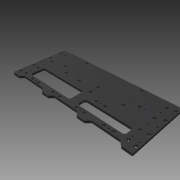
# Autodesk Inventor part: front
Saved by Autodesk Inventor 2014 (Build 180170000, 170)
## iProperties
Created: 2013-12-05
Part Number: front
Material: Plywood, Finish
Document SubType Name: Modeling
Designer: buben
Density: 0.552 g/cm^3
Appearance: Plywood - New
Author: buben
Subject: Laser Cutted
Autodesk Inventor part; units mm, degrees
ref_plane "YZ Plane" through (0, 0, 0) normal (1, 0, 0) x (0, 1, 0)
ref_plane "XZ Plane" through (0, 0, 0) normal (0, 1, 0) x (-1, 0, 0)
ref_plane "XY Plane" through (0, 0, 0) normal (0, 0, 1) x (1, 0, 0)
sketch "Sketch1" plane through (0, 0, 0) normal (0, 0, 1) x (1, 0, 0)
  line L0 (0, 0) -> (355, 0)
  line L1 (355, 0) -> (355, 150)
  line L2 (355, 150) -> (0, 150)
  line L3 (0, 150) -> (0, 0)
  dimension "d0" = 150
  dimension "d1" = 355
  constraints: 8 end point, 2 parallel, 1 horizontal, 1 perpendicular
  measures "d0" distance of L2.end L0.start
  measures "d1" distance of L0.start L0.end
extrude "Extrusion1" add sketch "Sketch1" along normal blind 6.5
sketch "Sketch3" plane through (0, 0, 6.5) normal (0, 0, 1) x (1, 0, 0)
  line L0 (0, 0) -> (355, 0) projected
  line L1 (355, 150) -> (0, 150) projected
  line L2 (0, 150) -> (0, 0) projected
  circle A0 centre (64.5, 96) radius 4
  circle A1 centre (290.5, 96) radius 4
  line L3 (64.5, 96) -> (290.5, 96) construction
  point P0 (177.5, 96)
  point P1 (177.5, 150)
  dimension "d9" = 8
  dimension "d10" = 96
  dimension "d11" = 226
  constraints: 2 centre point, 2 end point, 2 midpoint, 1 equal radius, 1 horizontal alignment, 1 perpendicular, 1 vertical alignment
  measures "d9" diameter of A0
  measures "d10" distance from line of L0 L3.start
  measures "d11" distance of L3.start L3.end
extrude "Extrusion3" cut sketch "Sketch3" against normal through all
sketch "Sketch4" plane through (0, 0, 6.5) normal (0, 0, 1) x (1, 0, 0)
  line L0 (0, 0) -> (355, 0) projected
  line L1 (355, 150) -> (0, 150) projected
  line L2 (0, 150) -> (0, 0) projected
  circle A0 centre (6.25, 18.5) radius 2.25
  circle A1 centre (6.25, 70.5) radius 2.25
  circle A2 centre (6.25, 122.5) radius 2.25
  line L3 (177.5, 150) -> (177.5, 0) construction
  line L4 (3, 138) -> (9.5, 138)
  line L5 (9.5, 138) -> (9.5, 130)
  line L6 (9.5, 130) -> (3, 130)
  line L7 (3, 130) -> (3, 138)
  line L8 (3, 100.5) -> (9.5, 100.5)
  line L9 (9.5, 100.5) -> (9.5, 92.5)
  line L10 (9.5, 92.5) -> (3, 92.5)
  line L11 (3, 92.5) -> (3, 100.5)
  line L12 (3, 48.5) -> (9.5, 48.5)
  line L13 (9.5, 48.5) -> (9.5, 40.5)
  line L14 (9.5, 40.5) -> (3, 40.5)
  line L15 (3, 40.5) -> (3, 48.5)
  line L16 (3, 11) -> (9.5, 11)
  line L17 (9.5, 11) -> (9.5, 3)
  line L18 (9.5, 3) -> (3, 3)
  line L19 (3, 3) -> (3, 11)
  line L20 (6.25, 18.5) -> (6.25, 70.5) construction
  line L21 (6.25, 70.5) -> (6.25, 122.5) construction
  circle A3 centre (348.75, 18.5) radius 2.25
  circle A4 centre (348.75, 70.5) radius 2.25
  circle A5 centre (348.75, 122.5) radius 2.25
  line L22 (352, 138) -> (345.5, 138)
  line L23 (345.5, 138) -> (345.5, 130)
  line L24 (345.5, 130) -> (352, 130)
  line L25 (352, 130) -> (352, 138)
  line L26 (352, 100.5) -> (345.5, 100.5)
  line L27 (345.5, 100.5) -> (345.5, 92.5)
  line L28 (345.5, 92.5) -> (352, 92.5)
  line L29 (352, 92.5) -> (352, 100.5)
  line L30 (352, 48.5) -> (345.5, 48.5)
  line L31 (345.5, 48.5) -> (345.5, 40.5)
  line L32 (345.5, 40.5) -> (352, 40.5)
  line L33 (352, 40.5) -> (352, 48.5)
  line L34 (352, 11) -> (345.5, 11)
  line L35 (345.5, 11) -> (345.5, 3)
  line L36 (345.5, 3) -> (352, 3)
  line L37 (352, 3) -> (352, 11)
  line L38 (348.75, 18.5) -> (348.75, 70.5) construction
  line L39 (348.75, 70.5) -> (348.75, 122.5) construction
  point P0 (6.25, 130)
  point P1 (3, 44.5)
  point P2 (6.25, 44.5)
  point P3 (3, 96.5)
  point P4 (6.25, 96.5)
  point P5 (348.75, 130)
  point P6 (352, 44.5)
  point P7 (348.75, 44.5)
  point P8 (352, 96.5)
  point P9 (348.75, 96.5)
  dimension "d14" = 18.5
  dimension "d15" = 52
  dimension "d16" = 52
  dimension "d17" = 4.5
  dimension "d18" = 6.5
  dimension "d19" = 8
  dimension "d20" = 8
  dimension "d21" = 8
  dimension "d22" = 8
  dimension "d28" = 3
  dimension "d90" = 7.5
  dimension "d91" = 7.5
  constraints: 74 end point, 24 symmetric about line, 9 parallel, 7 collinear, 7 midpoint, 6 centre point, 4 horizontal, 4 perpendicular, 3 vertical alignment, 2 equal radius, 2 horizontal alignment, 3 other
  measures "d14" distance from line of L0 L20.start
  measures "d15" distance of L20.start L20.end
  measures "d16" distance of L20.end L21.end
  measures "d17" diameter of A0
  measures "d18" distance of L4.start L4.end
  measures "d19" distance of L6.end L4.start
  measures "d20" distance of L10.end L8.start
  measures "d21" distance of L14.end L12.start
  measures "d22" distance of L18.end L16.start
  measures "d28" distance between parallel lines of L2 L7
  measures "d90" distance from line of L21.end L6
  measures "d91" distance from line of L20.start L16
extrude "Extrusion4" cut sketch "Sketch4" against normal through all
sketch "Sketch5" plane through (0, 0, 6.5) normal (0, 0, 1) x (1, 0, 0)
  line L0 (0, 0) -> (355, 0) projected
  line L1 (51, 9.5) -> (59, 9.5)
  line L2 (59, 9.5) -> (59, 3)
  line L3 (59, 3) -> (51, 3)
  line L4 (51, 3) -> (51, 9.5)
  line L5 (74, 9.5) -> (82, 9.5)
  line L6 (82, 9.5) -> (82, 3)
  line L7 (82, 3) -> (74, 3)
  line L8 (74, 3) -> (74, 9.5)
  line L9 (59, 9.5) -> (74, 3) construction
  line L10 (74, 9.5) -> (59, 3) construction
  circle A0 centre (66.5, 6.25) radius 2.25
  line L11 (125, 9.5) -> (133, 9.5)
  line L12 (133, 9.5) -> (133, 3)
  line L13 (133, 3) -> (125, 3)
  line L14 (125, 3) -> (125, 9.5)
  line L15 (148, 9.5) -> (156, 9.5)
  line L16 (156, 9.5) -> (156, 3)
  line L17 (156, 3) -> (148, 3)
  line L18 (148, 3) -> (148, 9.5)
  line L19 (133, 9.5) -> (148, 3) construction
  line L20 (148, 9.5) -> (133, 3) construction
  circle A1 centre (140.5, 6.25) radius 2.25
  line L21 (199, 9.5) -> (207, 9.5)
  line L22 (207, 9.5) -> (207, 3)
  line L23 (207, 3) -> (199, 3)
  line L24 (199, 3) -> (199, 9.5)
  line L25 (222, 9.5) -> (230, 9.5)
  line L26 (230, 9.5) -> (230, 3)
  line L27 (230, 3) -> (222, 3)
  line L28 (222, 3) -> (222, 9.5)
  line L29 (207, 9.5) -> (222, 3) construction
  line L30 (222, 9.5) -> (207, 3) construction
  circle A2 centre (214.5, 6.25) radius 2.25
  line L31 (273, 9.5) -> (281, 9.5)
  line L32 (281, 9.5) -> (281, 3)
  line L33 (281, 3) -> (273, 3)
  line L34 (273, 3) -> (273, 9.5)
  line L35 (296, 9.5) -> (304, 9.5)
  line L36 (304, 9.5) -> (304, 3)
  line L37 (304, 3) -> (296, 3)
  line L38 (296, 3) -> (296, 9.5)
  line L39 (281, 9.5) -> (296, 3) construction
  line L40 (296, 9.5) -> (281, 3) construction
  circle A3 centre (288.5, 6.25) radius 2.25
  line L41 (82, 6.25) -> (125, 6.25) construction
  line L42 (156, 6.25) -> (199, 6.25) construction
  line L43 (230, 6.25) -> (273, 6.25) construction
  line L44 (9.5, 11) -> (9.5, 3) projected
  line L45 (345.5, 3) -> (345.5, 11) projected
  point P0 (288.5, 6.25)
  dimension "d31" = 8
  dimension "d32" = 6.5
  dimension "d33" = 8
  dimension "d34" = 15
  dimension "d35" = 4.5
  dimension "d36" = 8
  dimension "d37" = 6.5
  dimension "d38" = 8
  dimension "d39" = 15
  dimension "d40" = 4.5
  dimension "d41" = 8
  dimension "d42" = 6.5
  dimension "d43" = 8
  dimension "d44" = 15
  dimension "d45" = 4.5
  dimension "d46" = 8
  dimension "d47" = 6.5
  dimension "d48" = 8
  dimension "d49" = 15
  dimension "d50" = 4.5
  dimension "d51" = 3
  dimension "d88" = 57
  dimension "d89" = 57
  constraints: 86 end point, 16 parallel, 11 midpoint, 10 collinear, 8 horizontal, 8 perpendicular, 4 centre point, 3 horizontal alignment
  measures "d31" distance of L1.start L1.end
  measures "d32" distance of L3.end L1.start
  measures "d33" distance of L5.start L5.end
  measures "d34" distance between parallel lines of L8 L2
  measures "d35" diameter of A0
  measures "d36" distance of L14.end L11.end
  measures "d37" distance of L14.start L14.end
  measures "d38" distance of L20.start L15.end
  measures "d39" distance between parallel lines of L18 L12
  measures "d40" diameter of A1
  measures "d41" distance of L24.end L21.end
  measures "d42" distance of L24.start L24.end
  measures "d43" distance of L30.start L25.end
  measures "d44" distance between parallel lines of L28 L22
  measures "d45" diameter of A2
  measures "d46" distance of L34.end L31.end
  measures "d47" distance of L34.start L34.end
  measures "d48" distance of L40.start L35.end
  measures "d49" distance between parallel lines of L38 L32
  measures "d50" diameter of A3
  measures "d51" distance between parallel lines of L0 L3
  measures "d88" distance from line of L44 A0.centre
  measures "d89" distance from line of L45 point (288.5, 6.25)
extrude "Extrusion5" cut sketch "Sketch5" against normal through all
sketch "Sketch6" plane through (0, 0, 6.5) normal (0, 0, 1) x (1, 0, 0)
  line L0 (0, 0) -> (355, 0) projected
  line L1 (0, 150) -> (0, 0) projected
  line L2 (0, 0) -> (0, -10)
  line L3 (0, -10) -> (23, -10)
  line L4 (23, -10) -> (33, 0)
  line L5 (102.6667, 0) -> (112.6667, -10)
  line L6 (112.6667, -10) -> (132.6667, -10)
  line L7 (132.6667, -10) -> (142.6667, 0)
  line L8 (212.3333, 0) -> (222.3333, -10)
  line L9 (222.3333, -10) -> (242.3333, -10)
  line L10 (242.3333, -10) -> (252.3333, 0)
  line L11 (355, 0) -> (355, -10)
  line L12 (355, -10) -> (332, -10)
  line L13 (332, -10) -> (322, 0)
  line L14 (23, -10) -> (112.6667, -10) construction
  line L15 (132.6667, -10) -> (222.3333, -10) construction
  line L16 (242.3333, -10) -> (332, -10) construction
  dimension "d54" = 20
  dimension "d55" = 23
  dimension "d56" = 45
  dimension "d57" = 10
  constraints: 30 end point, 13 collinear, 8 perpendicular, 6 point on line
  measures "d54" distance of L5.end L6.end
  measures "d55" distance of L2.end L3.end
  measures "d56" angle of L4 L3
  measures "d57" distance of L0.start L2.end
extrude "Extrusion6" add sketch "Sketch6" against normal blind 6.5
sketch "Sketch11" plane through (0, 0, 6.5) normal (0, 0, 1) x (1, 0, 0)
  line L0 (9.5, 138) -> (9.5, 130) projected
  line L1 (345.5, 130) -> (345.5, 138) projected
  line L2 (355, 150) -> (0, 150) projected
  line L3 (89.5, 147) -> (97.5, 147)
  line L4 (97.5, 147) -> (97.5, 140.5)
  line L5 (97.5, 140.5) -> (89.5, 140.5)
  line L6 (89.5, 140.5) -> (89.5, 147)
  line L7 (257.5, 147) -> (265.5, 147)
  line L8 (265.5, 147) -> (265.5, 140.5)
  line L9 (265.5, 140.5) -> (257.5, 140.5)
  line L10 (257.5, 140.5) -> (257.5, 147)
  point P0 (0, 0)
  dimension "d92" = 6.5
  dimension "d93" = 8
  dimension "d94" = 3
  dimension "d95" = 80
  dimension "d96" = 80
  constraints: 16 end point, 4 parallel, 3 collinear, 2 horizontal, 2 perpendicular
  measures "d92" distance of L5.end L3.start
  measures "d93" distance of L3.start L3.end
  measures "d94" distance between parallel lines of L2 L3
  measures "d95" distance between parallel lines of L0 L6
  measures "d96" distance between parallel lines of L1 L8
extrude "Extrusion11" cut sketch "Sketch11" against normal through all
chamfer "Chamfer1" distance 2 angle 45 4 edges at (355, -10, 3.25) (355, 150, 3.25) (0, -10, 3.25) (0, 150, 3.25)
sketch "Sketch12" plane through (0, 0, 6.5) normal (0, 0, 1) x (1, 0, 0)
  line L0 (51, 9.5) -> (59, 9.5) projected
  line L1 (9.5, 48.5) -> (9.5, 40.5) projected
  line L2 (86.5, 81) -> (94.5, 81)
  line L3 (94.5, 81) -> (94.5, 74.5)
  line L4 (94.5, 74.5) -> (86.5, 74.5)
  line L5 (86.5, 74.5) -> (86.5, 81)
  line L6 (260.5, 81) -> (268.5, 81)
  line L7 (268.5, 81) -> (268.5, 74.5)
  line L8 (268.5, 74.5) -> (260.5, 74.5)
  line L9 (260.5, 74.5) -> (260.5, 81)
  line L10 (345.5, 40.5) -> (345.5, 48.5) projected
  point P0 (0, 0)
  dimension "d102" = 6.5
  dimension "d103" = 8
  dimension "d104" = 65
  dimension "d105" = 77
  dimension "d109" = 77
  constraints: 16 end point, 4 parallel, 3 collinear, 2 horizontal, 2 perpendicular
  measures "d102" distance of L4.end L2.start
  measures "d103" distance of L2.start L2.end
  measures "d104" distance between parallel lines of L0 L4
  measures "d105" distance between parallel lines of L1 L5
  measures "d109" distance between parallel lines of L10 L7
extrude "Extrusion12" cut sketch "Sketch12" against normal through all
sketch "Sketch13" plane through (0, 0, 6.5) normal (0, 0, 1) x (1, 0, 0)
  circle A0 centre (64.5, 96) radius 4 projected
  circle A1 centre (290.5, 96) radius 4 projected
  circle A2 centre (52.5, 96) radius 2.25
  circle A3 centre (76.5, 96) radius 2.25
  circle A4 centre (278.5, 96) radius 2.25
  circle A5 centre (302.5, 96) radius 2.25
  point P0 (0, 0)
  dimension "d110" = 4.5
  dimension "d111" = 12
  dimension "d112" = 12
  dimension "d113" = 12
  dimension "d114" = 12
  constraints: 4 centre point, 4 horizontal alignment, 3 equal radius
  measures "d110" diameter of A3
  measures "d111" distance of A0.centre A2.centre
  measures "d112" distance of A3.centre A0.centre
  measures "d113" distance of A1.centre A4.centre
  measures "d114" distance of A1.centre A5.centre
extrude "Extrusion13" cut sketch "Sketch13" against normal through all contours A2 | A3 | A4 | A5
sketch "Sketch14" plane through (0, 0, 6.5) normal (0, 0, 1) x (1, 0, 0)
  line L0 (33, 0) -> (102.6667, 0) projected
  line L1 (142.6667, 0) -> (212.3333, 0) projected
  line L2 (353, 150) -> (2, 150) projected
  line L3 (21, 13.7) -> (27.5, 13.7)
  line L4 (27.5, 13.7) -> (27.5, 5.7)
  line L5 (27.5, 5.7) -> (21, 5.7)
  line L6 (21, 5.7) -> (21, 13.7)
  line L7 (21, 47.4625) -> (27.5, 47.4625)
  line L8 (27.5, 47.4625) -> (27.5, 39.4625)
  line L9 (27.5, 39.4625) -> (21, 39.4625)
  line L10 (21, 39.4625) -> (21, 47.4625)
  line L11 (21, 91.9875) -> (27.5, 91.9875)
  line L12 (27.5, 91.9875) -> (27.5, 83.9875)
  line L13 (27.5, 83.9875) -> (21, 83.9875)
  line L14 (21, 83.9875) -> (21, 91.9875)
  line L15 (21, 135.25) -> (27.5, 135.25)
  line L16 (27.5, 135.25) -> (27.5, 127.25)
  line L17 (27.5, 127.25) -> (21, 127.25)
  line L18 (21, 127.25) -> (21, 135.25)
  circle A0 centre (24.25, 21.2) radius 2.25
  circle A1 centre (24.25, 65.725) radius 2.25
  circle A2 centre (24.25, 110.25) radius 2.25
  line L19 (24.25, 110.25) -> (24.25, 65.725) construction
  line L20 (24.25, 21.2) -> (24.25, 65.725) construction
  line L21 (177.5, 150) -> (177.5, 0) construction
  line L22 (334, 13.7) -> (327.5, 13.7)
  line L23 (327.5, 13.7) -> (327.5, 5.7)
  line L24 (327.5, 5.7) -> (334, 5.7)
  line L25 (334, 5.7) -> (334, 13.7)
  line L26 (334, 47.4625) -> (327.5, 47.4625)
  line L27 (327.5, 47.4625) -> (327.5, 39.4625)
  line L28 (327.5, 39.4625) -> (334, 39.4625)
  line L29 (334, 39.4625) -> (334, 47.4625)
  line L30 (334, 91.9875) -> (327.5, 91.9875)
  line L31 (327.5, 91.9875) -> (327.5, 83.9875)
  line L32 (327.5, 83.9875) -> (334, 83.9875)
  line L33 (334, 83.9875) -> (334, 91.9875)
  line L34 (334, 135.25) -> (327.5, 135.25)
  line L35 (327.5, 135.25) -> (327.5, 127.25)
  line L36 (327.5, 127.25) -> (334, 127.25)
  line L37 (334, 127.25) -> (334, 135.25)
  circle A3 centre (330.75, 21.2) radius 2.25
  circle A4 centre (330.75, 65.725) radius 2.25
  circle A5 centre (330.75, 110.25) radius 2.25
  line L38 (22, 112.5) -> (26.5, 112.5) construction
  line L39 (26.5, 112.5) -> (26.5, 108) construction
  line L40 (26.5, 108) -> (22, 108) construction
  line L41 (22, 108) -> (22, 112.5) construction
  line L42 (24.25, 112.5) -> (24.25, 150) construction
  point P0 (0, 0)
  point P1 (24.25, 127.25)
  point P2 (21, 43.4625)
  point P3 (24.25, 43.4625)
  point P4 (21, 87.9875)
  point P5 (24.25, 87.9875)
  point P6 (21, 131.25)
  point P7 (330.75, 127.25)
  point P8 (334, 43.4625)
  point P9 (330.75, 43.4625)
  point P10 (334, 87.9875)
  point P11 (330.75, 87.9875)
  point P12 (334, 131.25)
  point P13 (22, 110.25)
  point P14 (24.25, 131.25)
  dimension "d117" = 8
  dimension "d118" = 6.5
  dimension "d120" = 4.5
  dimension "d121" = 7.5
  dimension "d122" = 39.75
  dimension "d123" = 150
  dimension "d126" = 21.2
  dimension "d127" = 4.5
  constraints: 80 end point, 25 symmetric about line, 11 midpoint, 11 parallel, 7 collinear, 6 centre point, 6 perpendicular, 5 equal length, 5 horizontal, 4 horizontal alignment, 4 vertical alignment, 2 equal radius, 1 point on line, 3 other
  measures "d117" distance of L17.end L15.start
  measures "d118" distance of L15.start L15.end
  measures "d120" diameter of A0
  measures "d121" distance from line of L3 L20.start
  measures "d122" distance from line of L2 L19.start
  measures "d123" distance between parallel lines of L21 L16
  measures "d126" distance from line of L0 L20.start
  measures "d127" distance of L39.end L40.end
extrude "Extrusion14" cut sketch "Sketch14" against normal through all
sketch "Sketch15" plane through (0, 0, 6.5) normal (0, 0, 1) x (1, 0, 0)
  line L0 (199, 9.5) -> (207, 9.5) projected
  line L1 (9.5, 48.5) -> (9.5, 40.5) projected
  line L2 (182.5, 90.99) -> (189, 90.99)
  line L3 (189, 90.99) -> (189, 82.99)
  line L4 (189, 82.99) -> (182.5, 82.99)
  line L5 (182.5, 82.99) -> (182.5, 90.99)
  line L6 (182.5, 67.99) -> (189, 67.99)
  line L7 (189, 67.99) -> (189, 59.99)
  line L8 (189, 59.99) -> (182.5, 59.99)
  line L9 (182.5, 59.99) -> (182.5, 67.99)
  circle A0 centre (185.75, 75.49) radius 2.25
  line L10 (214, 51.99) -> (222, 51.99)
  line L11 (222, 51.99) -> (222, 45.49)
  line L12 (222, 45.49) -> (214, 45.49)
  line L13 (214, 45.49) -> (214, 51.99)
  line L14 (237, 51.99) -> (245, 51.99)
  line L15 (245, 51.99) -> (245, 45.49)
  line L16 (245, 45.49) -> (237, 45.49)
  line L17 (237, 45.49) -> (237, 51.99)
  circle A1 centre (229.5, 48.74) radius 2.25
  point P0 (0, 0)
  point P1 (185.75, 82.99)
  point P2 (222, 48.74)
  dimension "d128" = 8
  dimension "d129" = 6.5
  dimension "d130" = 15
  dimension "d131" = 4.5
  dimension "d132" = 7.5
  dimension "d133" = 173
  dimension "d134" = 65.99
  dimension "d140" = 15
  dimension "d141" = 7.5
  dimension "d142" = 8
  dimension "d143" = 25
  constraints: 32 end point, 8 parallel, 4 collinear, 4 equal length, 4 horizontal, 4 perpendicular, 2 centre point, 2 midpoint, 1 equal radius, 1 horizontal alignment, 1 vertical alignment
  measures "d128" distance of L4.end L2.start
  measures "d129" distance of L2.start L2.end
  measures "d130" distance between parallel lines of L6 L4
  measures "d131" diameter of A0
  measures "d132" distance from line of L4 A0.centre
  measures "d133" distance between parallel lines of L1 L5
  measures "d134" distance from line of L0 A0.centre
  measures "d140" distance between parallel lines of L17 L11
  measures "d141" distance from line of L11 A1.centre
  measures "d142" distance between parallel lines of L8 L10
  measures "d143" distance between parallel lines of L13 L7
extrude "Extrusion15" cut sketch "Sketch15" against normal through all
sketch "Sketch16" plane through (0, 0, 6.5) normal (0, 0, 1) x (1, 0, 0)
  line L0 (182.5, 59.99) -> (182.5, 67.99) projected
  line L1 (189, 67.99) -> (189, 59.99) projected
  line L2 (245, 45.49) -> (237, 45.49) projected
  line L3 (327.5, 5.7) -> (327.5, 13.7) projected
  line L4 (27.5, 13.7) -> (27.5, 5.7) projected
  line L5 (74, 9.5) -> (82, 9.5) projected
  line L6 (39.5, 53.5) -> (170.5, 53.5)
  line L7 (174.5, 49.5) -> (174.5, 17.5)
  line L8 (170.5, 13.5) -> (39.5, 13.5)
  line L9 (35.5, 17.5) -> (35.5, 49.5)
  line L10 (201, 37.49) -> (315.5, 37.49)
  line L11 (319.5, 33.49) -> (319.5, 17.5)
  line L12 (315.5, 13.5) -> (201, 13.5)
  line L13 (197, 17.5) -> (197, 33.49)
  line L14 (35.5, 49.5) -> (39.5, 53.5)
  line L15 (35.5, 17.5) -> (39.5, 13.5)
  line L16 (170.5, 13.5) -> (174.5, 17.5)
  line L17 (174.5, 49.5) -> (170.5, 53.5)
  line L18 (197, 33.49) -> (201, 37.49)
  line L19 (315.5, 37.49) -> (319.5, 33.49)
  line L20 (319.5, 17.5) -> (315.5, 13.5)
  line L21 (201, 13.5) -> (197, 17.5)
  point P0 (0, 0)
  point P1 (35.5, 53.5)
  point P2 (174.5, 13.5)
  point P3 (174.5, 53.5)
  point P4 (35.5, 13.5)
  point P5 (197, 37.49)
  point P6 (319.5, 13.5)
  point P7 (319.5, 37.49)
  point P8 (197, 13.5)
  dimension "d146" = 4
  dimension "d147" = 4
  dimension "d148" = 4
  dimension "d149" = 4
  dimension "d150" = 4
  dimension "d151" = 4
  dimension "d152" = 4
  dimension "d153" = 4
  dimension "d154" = 4
  dimension "d155" = 4
  dimension "d156" = 4
  dimension "d157" = 4
  dimension "d158" = 4
  dimension "d159" = 4
  dimension "d160" = 4
  dimension "d161" = 4
  dimension "d162" = 4
  dimension "d163" = 8
  dimension "d164" = 8
  dimension "d165" = 8
  dimension "d166" = 8
  dimension "d167" = 8
  dimension "d168" = 40
  constraints: 32 end point, 16 point on line, 4 parallel, 2 horizontal, 2 perpendicular, 1 collinear
  measures "d146" distance of L9.end point (35.5, 53.5)
  measures "d147" distance of L6.start point (35.5, 53.5)
  measures "d148" distance of L9.start point (35.5, 13.5)
  measures "d149" distance of L8.end point (35.5, 13.5)
  measures "d150" distance of L8.start point (174.5, 13.5)
  measures "d151" distance of L7.end point (174.5, 13.5)
  measures "d152" distance of L7.start point (174.5, 53.5)
  measures "d153" distance of L6.end point (174.5, 53.5)
  measures "d154" distance of L13.end point (197, 37.49)
  measures "d155" distance of L10.start point (197, 37.49)
  measures "d156" distance of L10.end point (319.5, 37.49)
  measures "d157" distance of L11.start point (319.5, 37.49)
  measures "d158" distance of L11.end point (319.5, 13.5)
  measures "d159" distance of L12.start point (319.5, 13.5)
  measures "d160" distance of L12.end point (197, 13.5)
  measures "d161" distance of L13.start point (197, 13.5)
  measures "d162" distance between parallel lines of L5 L8
  measures "d163" distance between parallel lines of L4 L9
  measures "d164" distance between parallel lines of L0 L7
  measures "d165" distance between parallel lines of L13 L1
  measures "d166" distance between parallel lines of L3 L11
  measures "d167" distance between parallel lines of L10 L2
  measures "d168" distance between parallel lines of L8 L6
extrude "Extrusion16" cut sketch "Sketch16" against normal through all
sketch "Sketch17" plane through (0, 0, 6.5) normal (0, 0, 1) x (1, 0, 0)
  line L0 (27.5, 91.9875) -> (27.5, 83.9875) projected
  line L1 (353, 150) -> (2, 150) projected
  line L2 (134.25, 80) -> (140.75, 80)
  line L3 (140.75, 80) -> (140.75, 72)
  line L4 (140.75, 72) -> (134.25, 72)
  line L5 (134.25, 72) -> (134.25, 80)
  point P0 (0, 0)
  dimension "d171" = 8
  dimension "d172" = 6.5
  dimension "d173" = 70
  dimension "d174" = 106.75
  constraints: 8 end point, 2 parallel, 1 horizontal, 1 perpendicular
  measures "d171" distance of L4.end L2.start
  measures "d172" distance of L2.start L2.end
  measures "d173" distance between parallel lines of L1 L2
  measures "d174" distance between parallel lines of L0 L5
extrude "Extrusion17" cut sketch "Sketch17" against normal through all
equation "\"d16\" = d15"
equation "\"d89\" = d88"
body "Solid1"
